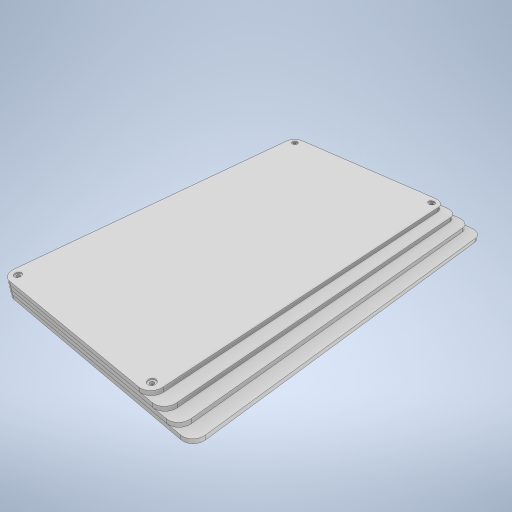
# Autodesk Inventor part: frame
Saved by Autodesk Inventor 2024 (Build 280153000, 153)
## iProperties
Created: 2023-10-17
Part Number: frame
Material: 常规
Document SubType Name: Modeling
Designer: Administrator
Density: 1 g/cm^3
Appearance: 默认
Author: Administrator
Autodesk Inventor part; units mm, degrees
ref_plane "YZ Plane" through (0, 0, 0) normal (1, 0, 0) x (0, 1, 0)
ref_plane "XY Plane" through (0, 0, 0) normal (0, 0, 1) x (1, 0, 0)
ref_plane "底层" through (0, -2, 0) normal (0, 1, 0) x (-1, 0, 0)
ref_plane "第二层" through (0, 4, 0) normal (0, 1, 0) x (-1, 0, 0)
ref_plane "第三层" through (0, 8, 0) normal (0, 1, 0) x (-1, 0, 0)
ref_plane "第四层" through (0, 12, 0) normal (0, 1, 0) x (-1, 0, 0)
sketch "底层草图" plane through (0, -2, 0) normal (0, 1, 0) x (-1, 0, 0)
  line L0 (-97, 140) -> (-97, -140)
  arc A0 (-97, -140) -> (-90, -147) centre (-90, -140) ccw
  line L1 (-90, -147) -> (90, -147)
  arc A1 (90, -147) -> (97, -140) centre (90, -140) ccw
  line L2 (97, -140) -> (97, 140)
  arc A2 (97, 140) -> (90, 147) centre (90, 140) ccw
  line L3 (90, 147) -> (-90, 147)
  arc A3 (-90, 147) -> (-97, 140) centre (-90, 140) ccw
  point P0 (0, 0)
  constraints: 8 end point, 8 point on circle, 4 centre point
sketch "第一层草图" plane through (0, 0, 0) normal (0, 1, 0) x (-1, 0, 0)
  line L0 (90, 150) -> (-90, 150)
  line L1 (-100, 140) -> (-100, -140)
  line L2 (-90, -150) -> (90, -150)
  line L3 (100, -140) -> (100, 140)
  line L4 (100, 150) -> (-100, -150) construction
  line L5 (-100, 150) -> (100, -150) construction
  arc A0 (100, 140) -> (90, 150) centre (90, 140) ccw
  arc A1 (-90, 150) -> (-100, 140) centre (-90, 140) ccw
  arc A2 (-100, -140) -> (-90, -150) centre (-90, -140) ccw
  arc A3 (90, -150) -> (100, -140) centre (90, -140) ccw
  point P0 (0, 0)
  dimension "d2" = 200
  dimension "d3" = 300
  dimension "d4" = 10
  constraints: 12 end point, 8 point on circle, 8 point on line, 8 tangent, 4 centre point, 3 equal radius, 2 midpoint, 2 parallel, 1 horizontal, 1 perpendicular
  measures "d2" distance of L5.end L4.end
  measures "d3" distance of L4.end L5.start
  measures "d4" radius of A0
sketch "第二层草图" plane through (0, 4, 0) normal (0, 1, 0) x (-1, 0, 0)
  line L0 (100, -140) -> (100, 140) projected
  line L1 (100, 0) -> (-88, 0)
  line L2 (90, 150) -> (-78, 150)
  line L3 (-88, 140) -> (-88, -140)
  line L4 (-78, -150) -> (90, -150)
  line L5 (100, -140) -> (100, 140)
  line L6 (100, 150) -> (-88, -150) construction
  line L7 (-88, 150) -> (100, -150) construction
  arc A0 (100, 140) -> (90, 150) centre (90, 140) ccw
  arc A1 (-78, 150) -> (-88, 140) centre (-78, 140) ccw
  arc A2 (-88, -140) -> (-78, -150) centre (-78, -140) ccw
  arc A3 (90, -150) -> (100, -140) centre (90, -140) ccw
  point P0 (0, 0)
  point P1 (6, 0)
  dimension "d101" = 188
  dimension "d102" = 188
  dimension "d103" = 300
  dimension "d104" = 10
  dimension "d125" = 10
  constraints: 14 end point, 8 point on circle, 8 point on line, 8 tangent, 4 centre point, 4 midpoint, 2 equal radius, 2 horizontal, 2 parallel, 1 perpendicular
  measures "d101" distance of L1.start L1.end
  measures "d102" distance of L7.end L6.end
  measures "d103" distance of L6.end L7.start
  measures "d104" radius of A0
  measures "d125" radius of A3
sketch "第三层草图" plane through (0, 8, 0) normal (0, 1, 0) x (-1, 0, 0)
  line L0 (100, -140) -> (100, 140) projected
  line L1 (100, 0) -> (-76, 0)
  line L2 (90, 150) -> (-66, 150)
  line L3 (-76, 140) -> (-76, -140)
  line L4 (-66, -150) -> (90, -150)
  line L5 (100, -140) -> (100, 140)
  line L6 (100, 150) -> (-76, -150) construction
  line L7 (-76, 150) -> (100, -150) construction
  arc A0 (100, 140) -> (90, 150) centre (90, 140) ccw
  arc A1 (-66, 150) -> (-76, 140) centre (-66, 140) ccw
  arc A2 (-76, -140) -> (-66, -150) centre (-66, -140) ccw
  arc A3 (90, -150) -> (100, -140) centre (90, -140) ccw
  point P0 (0, 0)
  point P1 (12, 0)
  dimension "d105" = 176
  dimension "d106" = 176
  dimension "d107" = 300
  dimension "d108" = 10
  constraints: 14 end point, 8 point on circle, 8 point on line, 8 tangent, 4 centre point, 4 midpoint, 3 equal radius, 2 horizontal, 2 parallel, 1 perpendicular
  measures "d105" distance of L1.start L1.end
  measures "d106" distance of L7.end L6.end
  measures "d107" distance of L6.end L7.start
  measures "d108" radius of A0
sketch "第四层草图" plane through (0, 12, 0) normal (0, 1, 0) x (-1, 0, 0)
  line L0 (100, -140) -> (100, 140) projected
  line L1 (100, 0) -> (-64, 0)
  line L2 (90, 150) -> (-54, 150)
  line L3 (-64, 140) -> (-64, -140)
  line L4 (-54, -150) -> (90, -150)
  line L5 (100, -140) -> (100, 140)
  line L6 (100, 150) -> (-64, -150) construction
  line L7 (-64, 150) -> (100, -150) construction
  arc A0 (100, 140) -> (90, 150) centre (90, 140) ccw
  arc A1 (-54, 150) -> (-64, 140) centre (-54, 140) ccw
  arc A2 (-64, -140) -> (-54, -150) centre (-54, -140) ccw
  arc A3 (90, -150) -> (100, -140) centre (90, -140) ccw
  point P0 (0, 0)
  point P1 (18, 0)
  dimension "d109" = 164
  dimension "d110" = 164
  dimension "d111" = 300
  dimension "d112" = 10
  dimension "d113" = 10
  constraints: 14 end point, 8 point on circle, 8 point on line, 8 tangent, 4 centre point, 4 midpoint, 2 equal radius, 2 horizontal, 2 parallel, 1 perpendicular
  measures "d109" distance of L1.start L1.end
  measures "d110" distance of L7.end L6.end
  measures "d111" distance of L6.end L7.start
  measures "d112" radius of A0
  measures "d113" radius of A2
extrude "拉伸25" add sketch "底层草图" along normal blind 2
extrude "拉伸26" add sketch "第一层草图" along normal blind 4 separate body
extrude "拉伸27" add sketch "第二层草图" along normal blind 4 separate body
extrude "拉伸28" add sketch "第三层草图" along normal blind 4 separate body
extrude "拉伸29" add sketch "第四层草图" along normal blind 4 separate body
sketch "草图20" plane through (0, 16, 0) normal (0, 1, 0) x (1, 0, 0)
  line L0 (-100, 140) -> (-100, -140) projected
  arc A0 (-100, -140) -> (-90, -150) centre (-90, -140) ccw projected
  line L1 (-90, -150) -> (54, -150) projected
  arc A1 (54, -150) -> (64, -140) centre (54, -140) ccw projected
  line L2 (64, -140) -> (64, 140) projected
  arc A2 (64, 140) -> (54, 150) centre (54, 140) ccw projected
  line L3 (54, 150) -> (-90, 150) projected
  arc A3 (-90, 150) -> (-100, 140) centre (-90, 140) ccw projected
  line L4 (-90, -140) -> (-92.1213, -142.1213)
  line L5 (-90, -140) -> (-87, -140) construction
  circle A4 centre (-92.1213, -142.1213) radius 2.75
  line L6 (-90, 140) -> (-92.1213, 142.1213)
  circle A5 centre (-92.1213, 142.1213) radius 2.75
  line L7 (54, -140) -> (56.1213, -142.1213)
  line L8 (54, -140) -> (57, -140) construction
  circle A6 centre (56.1213, -142.1213) radius 2.75
  line L9 (54, 140) -> (56.1213, 142.1213)
  circle A7 centre (56.1213, 142.1213) radius 2.75
  line L10 (-88, -138) -> (-88, 138)
  line L11 (-88, 138) -> (52, 138)
  line L12 (52, 138) -> (52, -138)
  line L13 (52, -138) -> (-88, -138)
  line L14 (-89.3713, -142.1213) -> (-90.7463, -144.5029)
  line L15 (-90.7463, -144.5029) -> (-93.4963, -144.5029)
  line L16 (-93.4963, -144.5029) -> (-94.8713, -142.1213)
  line L17 (-94.8713, -142.1213) -> (-93.4963, -139.7398)
  line L18 (-93.4963, -139.7398) -> (-90.7463, -139.7398)
  line L19 (-90.7463, -139.7398) -> (-89.3713, -142.1213)
  line L20 (-89.3713, 142.1213) -> (-90.7463, 139.7398)
  line L21 (-90.7463, 139.7398) -> (-93.4963, 139.7398)
  line L22 (-93.4963, 139.7398) -> (-94.8713, 142.1213)
  line L23 (-94.8713, 142.1213) -> (-93.4963, 144.5029)
  line L24 (-93.4963, 144.5029) -> (-90.7463, 144.5029)
  line L25 (-90.7463, 144.5029) -> (-89.3713, 142.1213)
  line L26 (58.8713, 142.1213) -> (57.4963, 139.7398)
  line L27 (57.4963, 139.7398) -> (54.7463, 139.7398)
  line L28 (54.7463, 139.7398) -> (53.3713, 142.1213)
  line L29 (53.3713, 142.1213) -> (54.7463, 144.5029)
  line L30 (54.7463, 144.5029) -> (57.4963, 144.5029)
  line L31 (57.4963, 144.5029) -> (58.8713, 142.1213)
  line L32 (58.8713, -142.1213) -> (57.4963, -144.5029)
  line L33 (57.4963, -144.5029) -> (54.7463, -144.5029)
  line L34 (54.7463, -144.5029) -> (53.3713, -142.1213)
  line L35 (53.3713, -142.1213) -> (54.7463, -139.7398)
  line L36 (54.7463, -139.7398) -> (57.4963, -139.7398)
  line L37 (57.4963, -139.7398) -> (58.8713, -142.1213)
  circle A8 centre (-92.1213, -142.1213) radius 1.6
  circle A9 centre (-92.1213, 142.1213) radius 1.6
  circle A10 centre (56.1213, -142.1213) radius 1.6
  circle A11 centre (56.1213, 142.1213) radius 1.6
  point P0 (0, 0)
  dimension "d128" = 5.5
  dimension "d130" = 5.5
  dimension "d132" = 5.5
  dimension "d134" = 5.5
  dimension "d126" = 3
  dimension "d127" = 135
  dimension "d129" = 3
  dimension "d131" = 45
  dimension "d133" = 3
  dimension "d135" = 12
  dimension "d136" = 3.2
  dimension "d137" = 3.2
  dimension "d138" = 3.2
  dimension "d139" = 3.2
  constraints: 68 end point, 12 coincident, 4 centre point, 4 horizontal alignment, 2 equal length, 2 horizontal, 63 other
  measures "d126" distance of L4.start L4.end
  measures "d127" angle of L4 L5
  measures "d129" distance of L6.start L6.end
  measures "d131" angle of L7 L8
  measures "d133" distance of L9.start L9.end
  measures "d135" distance between parallel lines of L0 L10
  measures "d136" diameter of A8
  measures "d137" diameter of A9
  measures "d138" diameter of A10
  measures "d139" diameter of A11
extrude "拉伸30" cut sketch "草图20" against normal up to surface (18 mm away) contours L10 L11 L12 L13 bodies 4 3 2
hole "四角固定孔" at (-92.1213, 16, 142.1213) at (-92.1213, 16, -142.1213) at (56.1213, 16, -142.1213) at (56.1213, 16, 142.1213) direction (0, -1, 0) diameter 3.2 end through all counterbore diameter 6.2 counterbore depth 1 bodies 5
extrude "六角通孔1" cut sketch "草图20" against normal through all contours L19 L14 L15 L16 L17 L18 | A8 bodies 4 3 2
extrude "六角通孔2" cut sketch "草图20" against normal through all contours L35 L36 L37 L32 L33 L34 | A10 bodies 4 3 2
extrude "六角通孔3" cut sketch "草图20" against normal through all contours L28 L29 L30 L31 L26 L27 | A11 bodies 4 3 2
extrude "六角通孔4" cut sketch "草图20" against normal through all contours L20 L21 L22 L23 L24 L25 | A9 bodies 4 3 2
sketch "底部孔草图" plane through (0, -2, 0) normal (0, -1, 0) x (1, 0, 0)
  circle A0 centre (-92.1213, -142.1213) radius 2.75 projected
  circle A1 centre (56.1213, -142.1213) radius 2.75 projected
  circle A2 centre (56.1213, 142.1213) radius 2.75 projected
  circle A3 centre (-92.1213, 142.1213) radius 2.75 projected
  point P0 (0, 0)
hole "孔2" at (-92.1213, -2, -142.1213) at (-92.1213, -2, 142.1213) at (56.1213, -2, 142.1213) at (56.1213, -2, -142.1213) direction (0, 1, 0) diameter 3.2 end through all counterbore diameter 6.2 counterbore depth 1 bodies 1
